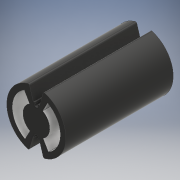
# Autodesk Inventor part: heatsink
Saved by Autodesk Inventor 2017 (Build 210142000, 142)
## iProperties
Created: 2018-04-04
Part Number: heatsink
Material: Generic
Document SubType Name: Modeling
Designer: dasae
Density: 1 g/cm^3
Appearance: Default
Author: dasae
Autodesk Inventor part; units mm, degrees
ref_plane "YZ Plane" through (0, 0, 0) normal (1, 0, 0) x (0, 1, 0)
ref_plane "XZ Plane" through (0, 0, 0) normal (0, 1, 0) x (-1, 0, 0)
ref_plane "XY Plane" through (0, 0, 0) normal (0, 0, 1) x (1, 0, 0)
sketch "Sketch3" plane through (0, 0, 0) normal (0, 1, 0) x (-1, 0, 0)
  arc A0 (1.0182, -10.1702) -> (-1.0182, -10.1702) centre (0, -9.4996) ccw
  arc A1 (-1.0182, 10.1702) -> (1.0182, 10.1702) centre (0, 9.4996) ccw
  arc A2 (4.8418, -19.4929) -> (6.015, -20.1262) centre (5.7451, -19.223) ccw
  line L0 (4.8418, -19.4929) -> (2.1573, -10.5106)
  arc A3 (-6.015, -20.1262) -> (-4.8418, -19.4929) centre (-5.7451, -19.223) ccw
  line L1 (-4.8418, -19.4929) -> (-2.1573, -10.5106)
  arc A4 (6.015, 20.1262) -> (4.8418, 19.4929) centre (5.7451, 19.223) ccw
  line L2 (4.8418, 19.4929) -> (2.1573, 10.5106)
  line L3 (-4.8418, 19.4929) -> (-2.1573, 10.5106)
  arc A5 (-4.8418, 19.4929) -> (-6.015, 20.1262) centre (-5.7451, 19.223) ccw
  arc A6 (-1.0182, 10.1702) -> (-2.1573, 10.5106) centre (-1.5824, 10.3585) ccw
  arc A7 (2.1573, 10.5106) -> (1.0182, 10.1702) centre (1.5824, 10.3585) ccw
  arc A8 (-2.1573, -10.5106) -> (-1.0182, -10.1702) centre (-1.5824, -10.3585) ccw
  arc A9 (1.0182, -10.1702) -> (2.1573, -10.5106) centre (1.5824, -10.3585) ccw
  arc A10 (-6.015, 20.1262) -> (-6.015, -20.1262) centre (0, 0) ccw
  arc A11 (6.015, -20.1262) -> (6.015, 20.1262) centre (0, 0) ccw
  line L4 (-8.0176, -15.13) -> (-4.448, -8.3939)
  line L5 (4.448, 8.3939) -> (8.0176, 15.13)
  line L6 (-4.7339, 8.236) -> (-8.5329, 14.8454)
  line L7 (4.7339, -8.236) -> (8.5329, -14.8454)
  arc A12 (-4.7339, 8.236) -> (-4.448, -8.3939) centre (0, 0) ccw
  arc A13 (4.7339, -8.236) -> (4.448, 8.3939) centre (0, 0) ccw
  arc A14 (8.5329, -14.8454) -> (8.0176, 15.13) centre (0, 0) ccw
  arc A15 (-8.5329, 14.8454) -> (-8.0176, -15.13) centre (0, 0) ccw
  point P0 (1.8035, -9.3268)
  point P1 (-1.8035, -9.3268)
  point P2 (1.8035, 9.3268)
  point P3 (-1.8035, 9.3268)
  dimension "d20" = 2.4384
  dimension "d21" = 2.4384
  constraints: 32 point on circle, 16 centre point, 16 end point, 2 coincident
  measures "d20" diameter of A0
  measures "d21" diameter of A1
extrude "Extrusion2" add sketch "Sketch3" along normal blind 76.2 contours A0 A8 L1 A3 A10 A5 L3 A6 A1 A7 L2 A4 A11 A2 L0 A9 | A15 L6 A12 L4 | L5 A14 L7 A13
sketch "Sketch4" plane through (0, 0, 0) normal (0, -1, 0) x (1, 0, 0)
  arc A0 (1.0182, -10.1702) -> (-1.0182, -10.1702) centre (0, -9.4996) ccw
  arc A1 (-1.0182, 10.1702) -> (1.0182, 10.1702) centre (0, 9.4996) ccw
  arc A2 (4.8418, -19.4929) -> (6.015, -20.1262) centre (5.7451, -19.223) ccw
  line L0 (4.8418, -19.4929) -> (2.1573, -10.5106)
  line L1 (-4.8418, -19.4929) -> (-2.1573, -10.5106)
  arc A3 (-6.015, -20.1262) -> (-4.8418, -19.4929) centre (-5.7451, -19.223) ccw
  line L2 (4.8418, 19.4929) -> (2.1573, 10.5106)
  arc A4 (6.015, 20.1262) -> (4.8418, 19.4929) centre (5.7451, 19.223) ccw
  line L3 (-4.8418, 19.4929) -> (-2.1573, 10.5106)
  arc A5 (-4.8418, 19.4929) -> (-6.015, 20.1262) centre (-5.7451, 19.223) ccw
  arc A6 (-1.0182, 10.1702) -> (-2.1573, 10.5106) centre (-1.5824, 10.3585) ccw
  arc A7 (2.1573, 10.5106) -> (1.0182, 10.1702) centre (1.5824, 10.3585) ccw
  arc A8 (1.0182, -10.1702) -> (2.1573, -10.5106) centre (1.5824, -10.3585) ccw
  arc A9 (-2.1573, -10.5106) -> (-1.0182, -10.1702) centre (-1.5824, -10.3585) ccw
  arc A10 (-6.015, 20.1262) -> (-6.015, -20.1262) centre (0, 0) ccw
  arc A11 (6.015, -20.1262) -> (6.015, 20.1262) centre (0, 0) ccw
  line L4 (-8.0176, -15.13) -> (-4.448, -8.3939)
  line L5 (4.448, 8.3939) -> (8.0176, 15.13)
  line L6 (-4.7339, 8.236) -> (-8.5329, 14.8454)
  line L7 (4.7339, -8.236) -> (8.5329, -14.8454)
  arc A12 (-4.7339, 8.236) -> (-4.448, -8.3939) centre (0, 0) ccw
  arc A13 (4.7339, -8.236) -> (4.448, 8.3939) centre (0, 0) ccw
  arc A14 (8.5329, -14.8454) -> (8.0176, 15.13) centre (0, 0) ccw
  arc A15 (-8.5329, 14.8454) -> (-8.0176, -15.13) centre (0, 0) ccw
  point P0 (1.8035, -9.3268)
  point P1 (-1.8035, -9.3268)
  point P2 (1.8035, 9.3268)
  point P3 (-1.8035, 9.3268)
  dimension "d25" = 2.4384
  dimension "d26" = 2.4384
  constraints: 32 point on circle, 16 centre point, 16 end point, 2 coincident
  measures "d25" diameter of A0
  measures "d26" diameter of A1
extrude "Extrusion3" cut sketch "Sketch4" against normal blind 76.2 contours A15 L6 A12 L4 | L5 A14 L7 A13
body "Solid2"
